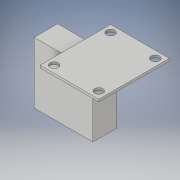
# Autodesk Inventor part: caster
Saved by Autodesk Inventor 2019 (Build 230136000, 136)
## iProperties
Created: 2018-09-07
Part Number: caster
Material: Generic
Document SubType Name: Modeling
Designer: mspet
Density: 1 g/cm^3
Appearance: Default
Author: mspet
Autodesk Inventor part; units mm, degrees
ref_plane "YZ Plane" through (0, 0, 0) normal (1, 0, 0) x (0, 1, 0)
ref_plane "XZ Plane" through (0, 0, 0) normal (0, 1, 0) x (-1, 0, 0)
ref_plane "XY Plane" through (0, 0, 0) normal (0, 0, 1) x (1, 0, 0)
sketch "Sketch1" plane through (0, 0, 0) normal (0, 1, 0) x (-1, 0, 0)
  line L0 (0, 0) -> (31.75, 0)
  line L1 (31.75, 0) -> (31.75, -38.1)
  line L2 (31.75, -38.1) -> (0, -38.1)
  line L3 (0, -38.1) -> (0, 0)
  dimension "d0" = 38.1
  dimension "d1" = 31.75
  constraints: 8 end point, 2 parallel, 1 horizontal, 1 perpendicular
  measures "d0" distance of L0.end L1.end
  measures "d1" distance of L1.end L2.end
extrude "Extrusion1" add sketch "Sketch1" along normal blind 1.27
sketch "Sketch2" plane through (0, 1.27, 0) normal (0, 1, 0) x (1, 0, 0)
  circle A0 centre (-27.94, 3.81) radius 2.2225
  line L0 (-31.75, 38.1) -> (-31.75, 0) projected
  line L1 (-31.75, 19.05) -> (0, 19.05) construction
  line L2 (-31.75, 0) -> (0, 0) projected
  line L3 (-15.875, 0) -> (-15.875, 38.1) construction
  line L4 (0, 38.1) -> (-31.75, 38.1) projected
  circle A1 centre (-27.94, 34.29) radius 2.2225
  circle A2 centre (-3.81, 3.81) radius 2.2225
  circle A3 centre (-3.81, 34.29) radius 2.2225
  point P0 (-15.875, 19.05)
  dimension "d4" = 3.81
  dimension "d5" = 3.81
  dimension "d6" = 4.445
  constraints: 4 centre point, 4 end point, 4 midpoint, 3 symmetric about line, 1 horizontal, 3 other
  measures "d4" distance from line of L0 A0.centre
  measures "d5" distance from line of L2 A0.centre
  measures "d6" diameter of A0
extrude "Extrusion2" cut sketch "Sketch2" against normal blind 1.27
sketch "Sketch3" plane through (0, 0, 0) normal (0, -1, 0) x (1, 0, 0)
  line L0 (-15.875, -25.4) -> (-15.875, -12.7)
  line L1 (-31.75, -38.1) -> (0, -38.1) projected
  line L2 (0, -38.1) -> (0, 0) projected
  line L3 (-15.875, -12.7) -> (-47.625, -12.7)
  line L4 (-47.625, -12.7) -> (-47.625, -25.4)
  line L5 (-47.625, -25.4) -> (-15.875, -25.4)
  line L6 (-15.875, -25.4) -> (-15.875, -12.7)
  dimension "d9" = 12.7
  dimension "d14" = 15.875
  dimension "d15" = 31.75
  constraints: 10 end point, 2 parallel, 1 horizontal, 1 perpendicular
  measures "d9" distance of L0.start L0.end
  measures "d14" distance between parallel lines of L2 L0
  measures "d15" distance of L4.end L5.end
extrude "Extrusion3" add sketch "Sketch3" along normal blind 33.02
body "Solid1"
